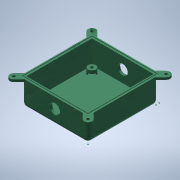
# Autodesk Inventor part: Base inferior
Saved by Autodesk Inventor 2021 (Build 250183000, 183)
## iProperties
Created: 2021-03-04
Part Number: Base inferior
Material: Steel, Mild, Welded
Document SubType Name: Modeling
Designer: Usuario
Density: 7.85 g/cm^3
Appearance: Smooth - Dark Sea Green
Author: Usuario
Autodesk Inventor part; units mm, degrees
ref_plane "YZ Plane" through (0, 0, 0) normal (1, 0, 0) x (0, 1, 0)
ref_plane "XZ Plane" through (0, 0, 0) normal (0, 1, 0) x (-1, 0, 0)
ref_plane "XY Plane" through (0, 0, 0) normal (0, 0, 1) x (1, 0, 0)
sketch "Sketch1" plane through (0, 0, 0) normal (0, 1, 0) x (-1, 0, 0)
  point P0 (0, 0)
sketch "Sketch2" plane through (0, 0, 0) normal (0, 1, 0) x (-1, 0, 0)
  line L0 (0, 0) -> (0, -90)
  line L1 (0, -90) -> (85, -90)
  line L2 (85, -90) -> (85, 0)
  line L3 (85, 0) -> (0, 0)
  dimension "d0" = 90
  dimension "d1" = 85
  constraints: 8 end point, 3 perpendicular, 1 vertical
  measures "d0" distance of L0.start L0.end
  measures "d1" distance of L0.end L1.end
extrude "Extrusion1" add sketch "Sketch2" along normal blind 3
sketch "Sketch3" plane through (0, 3, 0) normal (0, 1, 0) x (1, 0, 0)
  line L0 (0, 0) -> (0, 3)
  line L1 (0, 0) -> (0, 90) projected
  line L2 (0, 3) -> (0, 0)
  line L3 (-85, 90) -> (-85, 0) projected
  line L4 (0, 90) -> (-85, 90) projected
  line L5 (-3, 3) -> (-82, 3)
  line L6 (-82, 3) -> (-82, 87)
  line L7 (-82, 87) -> (-3, 87)
  line L8 (-3, 87) -> (-3, 3)
  line L9 (0, 90) -> (-85, 90) projected
  line L10 (-85, 0) -> (0, 0) projected
  line L11 (-85, 90) -> (0, 90)
  line L12 (0, 90) -> (0, 0)
  line L13 (0, 0) -> (-85, 0)
  line L14 (-85, 0) -> (-85, 90)
  constraints: 20 end point, 4 parallel, 2 horizontal, 2 perpendicular, 1 collinear, 1 point on line
extrude "Extrusion2" add sketch "Sketch3" along normal blind 30
sketch "Sketch7" plane through (-82, 3, -87) normal (0, 0, 1) x (1, 0, 0)
  point P0 (82, -3)
sketch "Sketch8" plane through (0, 33, 0) normal (0, 1, 0) x (1, 0, 0)
  line L0 (-3, 3) -> (-3, 87) projected
  line L1 (-3, 87) -> (-82, 87) projected
  line L2 (-82, 87) -> (-82, 3) projected
  line L3 (-82, 3) -> (-3, 3) projected
  line L4 (0, 0) -> (0, 90) projected
  line L5 (0, 90) -> (-85, 90) projected
  line L6 (-85, 90) -> (-85, 0) projected
  line L7 (-85, 0) -> (0, 0) projected
  line L8 (-3, 3) -> (-82, 3) projected
  line L9 (-82, 3) -> (-82, 87) projected
  line L10 (-82, 87) -> (-3, 87) projected
  line L11 (-3, 87) -> (-3, 3) projected
  line L12 (-85, 90) -> (-85, 0) projected
  line L13 (0, 0) -> (0, 90) projected
  line L14 (-85, 90) -> (0, 90)
  line L15 (0, 90) -> (0, 0)
  line L16 (0, 0) -> (-85, 0)
  line L17 (-85, 0) -> (-85, 90)
  line L18 (0, 90) -> (-85, 90) projected
  line L19 (-85, 91.5) -> (-86.5, 91.5)
  line L20 (0, -1.5) -> (1.5, -1.5)
  line L21 (-86.5, 91.5) -> (1.5, 91.5)
  line L22 (1.5, 91.5) -> (1.5, -1.5)
  line L23 (1.5, -1.5) -> (-86.5, -1.5)
  line L24 (-86.5, -1.5) -> (-86.5, 91.5)
  dimension "d26" = 1.5
  dimension "d27" = 1.5
  dimension "d28" = 1.5
  dimension "d29" = 1.5
  constraints: 20 end point, 4 parallel, 2 horizontal, 2 perpendicular, 1 point on line
  measures "d26" distance of L5.end L19.start
  measures "d27" distance of L19.start L19.end
  measures "d28" distance of L4.start L20.start
  measures "d29" distance of L20.start L20.end
extrude "Extrusion5" add sketch "Sketch8" against normal blind 3 contours L21 L22 L20 L23 L24 L19
sketch "Sketch9" plane through (0, 33, 0) normal (0, 1, 0) x (1, 0, 0)
  line L0 (-3, 3) -> (-3, 87) projected
  line L1 (-3, 87) -> (-82, 87) projected
  line L2 (-82, 87) -> (-82, 3) projected
  line L3 (-82, 3) -> (-3, 3) projected
  line L4 (1.5, 91.5) -> (-86.5, 91.5) projected
  line L5 (-86.5, 91.5) -> (-86.5, -1.5) projected
  line L6 (-86.5, -1.5) -> (1.5, -1.5) projected
  line L7 (1.5, -1.5) -> (1.5, 91.5) projected
  line L8 (-3, 3) -> (-82, 3) projected
  line L9 (-82, 3) -> (-82, 87) projected
  line L10 (-82, 87) -> (-3, 87) projected
  line L11 (-3, 87) -> (-3, 3) projected
  line L12 (-82, 3) -> (-82, 87) projected
  line L13 (-82, 87) -> (-82, 88.5)
  line L14 (-82, 88.5) -> (-83.5, 88.5)
  line L15 (-3, 87) -> (-3, 3) projected
  line L16 (-3, 3) -> (-1.5, 3)
  line L17 (-1.5, 3) -> (-1.5, 1.5)
  line L18 (-1.5, 1.5) -> (-83.5, 1.5)
  line L19 (-83.5, 1.5) -> (-83.5, 88.5)
  line L20 (-83.5, 88.5) -> (-1.5, 88.5)
  line L21 (-1.5, 88.5) -> (-1.5, 1.5)
  line L22 (-83.5, 88.5) -> (-83.5, 90)
  line L23 (0, 90) -> (-85, 90) projected
  line L24 (-83.5, 90) -> (-85, 90)
  line L25 (0, 0) -> (0, 90) projected
  line L26 (0, 0) -> (-85, 0)
  line L27 (-85, 0) -> (-85, 90)
  line L28 (-85, 90) -> (0, 90)
  line L29 (0, 90) -> (0, 0)
  dimension "d33" = 1.5
  dimension "d34" = 1.5
  dimension "d35" = 1.5
  dimension "d36" = 1.5
  dimension "d37" = 1.5
  constraints: 28 end point, 5 perpendicular, 4 parallel, 3 horizontal, 1 collinear, 1 point on line
  measures "d33" distance of L1.end L13.end
  measures "d34" distance of L13.end L14.end
  measures "d35" distance of L0.start L16.end
  measures "d36" distance of L16.end L17.end
  measures "d37" distance of L14.end L22.end
extrude "Extrusion6" cut sketch "Sketch9" against normal blind 0.7 contours L23 L25 L26 L27
sketch "Sketch10" plane through (-82, 3, -87) normal (0, 0, 1) x (1, 0, 0)
  line L0 (0, 30) -> (79, 30)
  line L1 (79, 30) -> (79, 0)
  line L2 (79, 0) -> (0, 0)
  line L3 (0, 0) -> (0, 30)
  line L4 (0, 30) -> (79, 30) projected
  line L5 (79, 0) -> (0, 0) projected
  circle A0 centre (39.5, 15) radius 6.4
  point P0 (82, -3)
  dimension "d40" = 12.8
  constraints: 8 end point, 2 parallel, 1 centre point, 1 horizontal, 1 perpendicular
  measures "d40" diameter of A0
extrude "Extrusion7" cut sketch "Sketch10" against normal blind 3 contours A0
sketch "Sketch11" plane through (-3, 3, -3) normal (0, 0, -1) x (-1, 0, 0)
  line L0 (0, 30) -> (79, 30) projected
  line L1 (79, 0) -> (0, 0)
  line L2 (0, 0) -> (0, 30)
  line L3 (0, 30) -> (79, 30)
  line L4 (79, 30) -> (79, 0)
  line L5 (79, 30) -> (0, 0)
  line L6 (79, 0) -> (0, 0) projected
  line L7 (0, 30) -> (79, 0)
  circle A0 centre (39.5, 15) radius 6.5
  point P0 (-3, -3)
  dimension "d43" = 13
  constraints: 12 end point, 2 parallel, 1 centre point, 1 horizontal, 1 midpoint, 1 perpendicular
  measures "d43" diameter of A0
extrude "Extrusion8" cut sketch "Sketch11" against normal blind 3 contours A0 L5 L7 | L7 L5 A0 | A0 L7 L5 | L5 L7 A0
sketch "Sketch12" plane through (0, 3, 0) normal (0, 1, 0) x (1, 0, 0)
  line L0 (-3, 3) -> (-3, 87) projected
  line L1 (-3, 87) -> (-82, 87) projected
  line L2 (-82, 87) -> (-82, 3) projected
  line L3 (-82, 3) -> (-3, 3) projected
  line L4 (-3, 87) -> (-3, 3) projected
  line L5 (-3, 3) -> (-82, 3) projected
  line L6 (-82, 87) -> (-3, 87) projected
  line L7 (-71.9395, 76.9395) -> (-13.0605, 13.0605) construction
  line L8 (-13.0605, 76.9395) -> (-71.9395, 13.0605) construction
  circle A0 centre (-13.0605, 13.0605) radius 5
  circle A1 centre (-13.0605, 76.9395) radius 5
  circle A2 centre (-71.9395, 76.9395) radius 5
  line L9 (-66.9395, 13.0605) -> (-62.9395, 13.0605) construction
  circle A3 centre (-71.9395, 13.0605) radius 5
  point P0 (0, 0)
  point P1 (-42.5, 45)
  dimension "d60" = 10
  dimension "d61" = 10
  dimension "d62" = 10
  dimension "d65" = 10
  constraints: 6 end point, 4 centre point, 4 coincident, 2 midpoint, 1 horizontal
  measures "d60" diameter of A0
  measures "d61" diameter of A1
  measures "d62" diameter of A2
  measures "d65" diameter of A3
extrude "Extrusion10" add sketch "Sketch12" along normal blind 4 contours A0 | A1 | A2 | A3
sketch "Sketch14" plane through (-71.9395, 7, -13.0605) normal (0, 1, 0) x (1, 0, 0)
  circle A0 centre (0, 0) radius 5 projected
  circle A1 centre (0, 63.879) radius 5 projected
  circle A2 centre (58.879, 0) radius 5 projected
  circle A3 centre (58.879, 63.879) radius 5 projected
  circle A4 centre (0, 0) radius 5 projected
  circle A5 centre (0, 0) radius 5
  circle A6 centre (0, 63.879) radius 5 projected
  circle A7 centre (0, 63.879) radius 5
  circle A8 centre (58.879, 63.879) radius 5
  circle A9 centre (58.879, 0) radius 5
  line L0 (0, 0) -> (-3.5355, 3.5355)
  line L1 (0, 0) -> (5, 0) construction
  line L2 (-3.5355, 3.5355) -> (3.5355, -3.5355)
  line L3 (0, 63.879) -> (-3.5355, 60.3435)
  line L4 (-3.5355, 60.3435) -> (3.5355, 67.4145)
  line L5 (58.879, 63.879) -> (55.3435, 67.4145)
  circle A10 centre (58.879, 63.879) radius 5 projected
  line L6 (55.3435, 67.4145) -> (62.4145, 60.3435)
  line L7 (58.879, 0) -> (55.3435, -3.5355)
  circle A11 centre (58.879, 0) radius 5 projected
  line L8 (55.3435, -3.5355) -> (62.4145, 3.5355)
  point P0 (71.9395, -13.0605)
  point P1 (62.4145, 3.5355)
  point P2 (3.5355, 67.4145)
  point P3 (-3.5355, 60.3435)
  point P4 (3.5355, -3.5355)
  point P5 (-3.5355, 3.5355)
  dimension "d68" = 135
  constraints: 18 end point, 4 coincident, 4 point on circle, 3 point on line, 2 centre point, 2 perpendicular, 1 equal length, 1 horizontal, 12 other
  measures "d68" angle of L1 L0
extrude "Extrusion11" cut sketch "Sketch14" against normal blind 4 contours A0 L2 L0 | A1 L3 L4 | L8 L7 A2 | L5 L6 A3 picked at (2.7524, 1.8391) picked at (3.1056, 62.7333) picked at (57.1671, 2.8318) picked at (55.576, 63.6792)
sketch "Sketch15" plane through (0, 7, 0) normal (0, 1, 0) x (1, 0, 0)
  line L0 (-68.404, 9.525) -> (-75.475, 16.596) projected
  arc A0 (-75.475, 16.596) -> (-68.404, 9.525) centre (-71.9395, 13.0605) ccw projected
  line L1 (-75.475, 73.404) -> (-68.404, 80.475) projected
  arc A1 (-68.404, 80.475) -> (-75.475, 73.404) centre (-71.9395, 76.9395) ccw projected
  line L2 (-16.596, 80.475) -> (-9.525, 73.404) projected
  arc A2 (-9.525, 73.404) -> (-16.596, 80.475) centre (-13.0605, 76.9395) ccw projected
  line L3 (-9.525, 16.596) -> (-16.596, 9.525) projected
  arc A3 (-16.596, 9.525) -> (-9.525, 16.596) centre (-13.0605, 13.0605) ccw projected
  circle A4 centre (-71.9395, 13.0605) radius 3.5
  circle A5 centre (-71.9395, 76.9395) radius 3.5
  circle A6 centre (-13.0605, 76.9395) radius 3.5
  circle A7 centre (-13.0605, 13.0605) radius 3.5
  point P0 (0, 0)
  dimension "d71" = 7
  dimension "d72" = 7
  dimension "d73" = 7
  dimension "d74" = 7
  constraints: 4 centre point, 4 coincident
  measures "d71" diameter of A4
  measures "d72" diameter of A5
  measures "d73" diameter of A6
  measures "d74" diameter of A7
extrude "Extrusion12" cut sketch "Sketch15" against normal blind 4 contours A4 L0 | L0 A4 | A5 L1 | L1 A5 | A6 L2 | L2 A6 | A7 L3 | L3 A7
sketch "Sketch16" plane through (0, 7, 0) normal (0, 1, 0) x (1, 0, 0)
  arc A0 (-74.4144, 15.5354) -> (-69.4646, 10.5856) centre (-71.9395, 13.0605) ccw projected
  line L0 (-74.4144, 15.5354) -> (-75.475, 16.596) projected
  arc A1 (-75.475, 16.596) -> (-68.404, 9.525) centre (-71.9395, 13.0605) ccw projected
  line L1 (-68.404, 9.525) -> (-69.4646, 10.5856) projected
  arc A2 (-15.5354, 10.5856) -> (-10.5856, 15.5354) centre (-13.0605, 13.0605) ccw projected
  line L2 (-15.5354, 10.5856) -> (-16.596, 9.525) projected
  arc A3 (-16.596, 9.525) -> (-9.525, 16.596) centre (-13.0605, 13.0605) ccw projected
  line L3 (-9.525, 16.596) -> (-10.5856, 15.5354) projected
  arc A4 (-10.5856, 74.4646) -> (-15.5354, 79.4144) centre (-13.0605, 76.9395) ccw projected
  line L4 (-10.5856, 74.4646) -> (-9.525, 73.404) projected
  arc A5 (-9.525, 73.404) -> (-16.596, 80.475) centre (-13.0605, 76.9395) ccw projected
  line L5 (-16.596, 80.475) -> (-15.5354, 79.4144) projected
  arc A6 (-69.4646, 79.4144) -> (-74.4144, 74.4646) centre (-71.9395, 76.9395) ccw projected
  line L6 (-69.4646, 79.4144) -> (-68.404, 80.475) projected
  arc A7 (-68.404, 80.475) -> (-75.475, 73.404) centre (-71.9395, 76.9395) ccw projected
  line L7 (-75.475, 73.404) -> (-74.4144, 74.4646) projected
  circle A8 centre (-71.9395, 13.0605) radius 5
  arc A9 (-68.404, 80.475) -> (-75.475, 73.404) centre (-71.9395, 76.9395) ccw projected
  circle A10 centre (-71.9395, 76.9395) radius 5
  circle A11 centre (-13.0605, 76.9395) radius 5
  circle A12 centre (-13.0605, 13.0605) radius 5
  point P0 (0, 0)
  point P1 (-75.475, 73.404)
  point P2 (-16.596, 80.475)
  point P3 (-68.404, 9.525)
  point P4 (-9.525, 16.596)
  constraints: 4 centre point, 4 coincident, 1 concentric
extrude "Extrusion13" add sketch "Sketch16" along normal blind 4
sketch "Sketch17" plane through (-13.0605, 11, -76.9395) normal (0, 1, 0) x (1, 0, 0)
  circle A0 centre (0, 0) radius 5 projected
  circle A1 centre (0, -63.879) radius 5 projected
  circle A2 centre (-58.879, 0) radius 5 projected
  circle A3 centre (-58.879, -63.879) radius 5 projected
  circle A4 centre (0, 0) radius 1.75
  arc A5 (3.5355, -60.3435) -> (-3.5355, -67.4145) centre (0, -63.879) ccw projected
  circle A6 centre (0, -63.879) radius 1.75
  circle A7 centre (-58.879, -63.879) radius 1.75
  circle A8 centre (-58.879, 0) radius 5 projected
  circle A9 centre (-58.879, 0) radius 1.75
  point P0 (13.0605, -76.9395)
  dimension "d79" = 3.5
  dimension "d80" = 3.5
  dimension "d81" = 3.5
  dimension "d82" = 3.5
  constraints: 4 centre point, 4 coincident
  measures "d79" diameter of A4
  measures "d80" diameter of A6
  measures "d81" diameter of A7
  measures "d82" diameter of A9
extrude "Extrusion14" cut sketch "Sketch17" against normal blind 4 contours A4 | A6 | A7 | A9
sketch "Sketch18" plane through (1.5, 33, -91.5) normal (0, 0, -1) x (-1, 0, 0)
  point P0 (1.5, -33)
sketch "Sketch20" plane through (0, 33, 0) normal (0, 1, 0) x (1, 0, 0)
  line L0 (1.5, 91.5) -> (1.5, -1.5) projected
  line L1 (1.5, -1.5) -> (5.0355, -5.0355)
  line L2 (1.5, -1.5) -> (6.5, -1.5) construction
  circle A0 centre (5.0355, -5.0355) radius 5
  line L3 (5.0355, -5.0355) -> (8.5711, -1.5)
  line L4 (8.5711, -1.5) -> (1.5, -8.5711)
  line L5 (1.5, -8.5711) -> (-5.5711, -1.5)
  line L6 (1.5, -1.5) -> (-86.5, -1.5) projected
  line L7 (8.5711, -1.5) -> (1.5, 5.5711)
  line L8 (-86.5, 91.5) -> (-86.5, -1.5) projected
  line L9 (-86.5, -1.5) -> (-90.0355, -5.0355)
  line L10 (-86.5, -1.5) -> (-81.5, -1.5) construction
  circle A1 centre (-90.0355, -5.0355) radius 5
  line L11 (-90.0355, -5.0355) -> (-86.5, -8.5711)
  line L12 (-86.5, -8.5711) -> (-93.5711, -1.5)
  line L13 (-93.5711, -1.5) -> (-86.5, 5.5711)
  line L14 (-86.5, -8.5711) -> (-79.4289, -1.5)
  line L15 (-86.5, 91.5) -> (-90.0355, 95.0355)
  line L16 (-86.5, 91.5) -> (-81.5, 91.5) construction
  circle A2 centre (-90.0355, 95.0355) radius 5
  line L17 (-90.0355, 95.0355) -> (-93.5711, 91.5)
  line L18 (-93.5711, 91.5) -> (-86.5, 98.5711)
  line L19 (-93.5711, 91.5) -> (-86.5, 84.4289)
  line L20 (-86.5, 98.5711) -> (-79.4289, 91.5)
  line L21 (-86.5, 91.5) -> (1.5, 91.5) projected
  line L22 (1.5, 91.5) -> (5.0355, 95.0355)
  line L23 (1.5, 91.5) -> (6.5, 91.5) construction
  circle A3 centre (5.0355, 95.0355) radius 5
  line L24 (5.0355, 95.0355) -> (8.5711, 91.5)
  line L25 (8.5711, 91.5) -> (1.5, 98.5711)
  line L26 (1.5, 98.5711) -> (-5.5711, 91.5)
  line L27 (8.5711, 91.5) -> (1.5, 84.4289)
  point P0 (0, 0)
  dimension "d85" = 5
  dimension "d86" = 45
  dimension "d87" = 5
  dimension "d88" = 135
  dimension "d89" = 5
  dimension "d90" = 135
  dimension "d91" = 5
  dimension "d92" = 45
  constraints: 48 end point, 12 point on line, 11 point on circle, 4 centre point, 4 coincident, 4 equal length, 4 horizontal, 4 parallel, 4 perpendicular, 4 tangent
  measures "d85" distance of L0.end L1.end
  measures "d86" angle of L1 L2
  measures "d87" distance of L6.end L9.end
  measures "d88" angle of L9 L10
  measures "d89" distance of L8.start L15.end
  measures "d90" angle of L16 L15
  measures "d91" distance of L0.start L22.end
  measures "d92" angle of L23 L22
extrude "Extrusion15" add sketch "Sketch20" against normal blind 3 contours A3 L27 L0 | A3 L25 L22 | L21 L26 A3 | L22 L24 A3 | L25 A3 L24 | L7 A0 L0 | L21 A2 L20 | A0 L3 L1 | L1 L4 A0 | A0 L5 L6 | A0 L4 L3 | L18 L17 A2 | A2 L15 L18 | A2 L17 L15 | L8 L19 A2 | L14 A1 L6 | L8 A1 L13 | A1 L11 L9 | L9 L12 A1 | A1 L12 L11
sketch "Sketch21" plane through (0, 33, 0) normal (0, 1, 0) x (1, 0, 0)
  line L0 (-5.5711, 91.5) -> (-79.4289, 91.5) projected
  line L1 (-79.4289, 91.5) -> (-86.5, 98.5711) projected
  arc A0 (-86.5, 98.5711) -> (-93.5711, 91.5) centre (-90.0355, 95.0355) ccw projected
  line L2 (-93.5711, 91.5) -> (-86.5, 84.4289) projected
  line L3 (-86.5, 84.4289) -> (-86.5, 5.5711) projected
  line L4 (-86.5, 5.5711) -> (-93.5711, -1.5) projected
  arc A1 (-93.5711, -1.5) -> (-86.5, -8.5711) centre (-90.0355, -5.0355) ccw projected
  line L5 (-86.5, -8.5711) -> (-79.4289, -1.5) projected
  line L6 (-79.4289, -1.5) -> (-5.5711, -1.5) projected
  line L7 (-5.5711, -1.5) -> (1.5, -8.5711) projected
  arc A2 (1.5, -8.5711) -> (8.5711, -1.5) centre (5.0355, -5.0355) ccw projected
  line L8 (8.5711, -1.5) -> (1.5, 5.5711) projected
  line L9 (1.5, 5.5711) -> (1.5, 84.4289) projected
  line L10 (1.5, 84.4289) -> (8.5711, 91.5) projected
  arc A3 (8.5711, 91.5) -> (1.5, 98.5711) centre (5.0355, 95.0355) ccw projected
  line L11 (1.5, 98.5711) -> (-5.5711, 91.5) projected
  line L12 (0, 0) -> (-85, 0) projected
  line L13 (-85, 0) -> (-85, 90) projected
  line L14 (-85, 90) -> (0, 90) projected
  line L15 (0, 90) -> (0, 0) projected
  circle A4 centre (5.0355, -5.0355) radius 1.75
  circle A5 centre (5.0355, 95.0355) radius 1.75
  circle A6 centre (-90.0355, 95.0355) radius 1.75
  circle A7 centre (-90.0355, -5.0355) radius 1.75
  dimension "d95" = 3.5
  dimension "d96" = 3.5
  dimension "d97" = 3.5
  dimension "d98" = 3.5
  constraints: 4 centre point, 4 coincident
  measures "d95" diameter of A4
  measures "d96" diameter of A5
  measures "d97" diameter of A6
  measures "d98" diameter of A7
extrude "Extrusion16" cut sketch "Sketch21" against normal blind 3 contours A4 | A5 | A6 | A7
fillet "Fillet1" radius 5 8 edges at (-85, 15, -90) (-85, 0, -45) (-42.5, 0, -90) (0, 15, -90) (0, 0, -45) (-42.5, 0, 0) (-85, 15, 0) (0, 15, 0)
body "Solid1"
